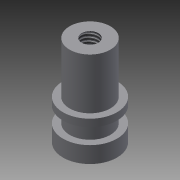
# Autodesk Inventor part: peek-insulator
Saved by Autodesk Inventor 2014 (Build 180170000, 170)
## iProperties
Created: 2013-12-31
Part Number: peek-insulator
Material: Generic
Document SubType Name: Modeling
Designer: caleb
Density: 1 g/cm^3
Appearance: Default
Author: caleb
Autodesk Inventor part; units mm, degrees
ref_plane "YZ Plane" through (0, 0, 0) normal (1, 0, 0) x (0, 1, 0)
ref_plane "XZ Plane" through (0, 0, 0) normal (0, 1, 0) x (-1, 0, 0)
ref_plane "XY Plane" through (0, 0, 0) normal (0, 0, 1) x (1, 0, 0)
sketch "Sketch1" plane through (0, 0, 0) normal (0, 0, 1) x (1, 0, 0)
  circle A0 centre (0, 0) radius 7.95
  dimension "d0" = 15.9
  constraints: 1 centre point, 1 coincident
  measures "d0" diameter of A0
extrude "Extrusion1" add sketch "Sketch1" along normal blind 4.82
sketch "Sketch2" plane through (0, 0, 4.82) normal (0, 0, 1) x (1, 0, 0)
  circle A0 centre (0, 0) radius 7.95 projected
  circle A1 centre (0, 0) radius 6
  dimension "d3" = 12
  constraints: 1 centre point, 1 coincident
  measures "d3" diameter of A1
extrude "Extrusion2" add sketch "Sketch2" along normal blind 4.6 contours A1
sketch "Sketch3" plane through (0, 0, 9.42) normal (0, 0, 1) x (1, 0, 0)
  circle A0 centre (0, 0) radius 6 projected
  circle A1 centre (0, 0) radius 7.95
  circle A2 centre (0, 0) radius 7.95 projected
  constraints: 1 centre point, 1 coincident, 1 concentric
extrude "Extrusion3" add sketch "Sketch3" along normal blind 2.15 contours A0 | A1
sketch "Sketch4" plane through (0, 0, 11.57) normal (0, 0, 1) x (1, 0, 0)
  circle A0 centre (0, 0) radius 7.95 projected
  circle A1 centre (0, 0) radius 6
  dimension "d8" = 12
  constraints: 1 centre point, 1 coincident
  measures "d8" diameter of A1
extrude "Extrusion4" add sketch "Sketch4" along normal blind 15 contours A1
sketch "Sketch5" plane through (0, 0, 0) normal (0, 0, -1) x (-1, 0, 0)
  circle A0 centre (0, 0) radius 7.95 projected
  constraints: 1 coincident
hole "Hole1" at (0, 0, 0) direction (0, 0, 1) diameter 4.917 end through all thread size "M6x1" class "6H" standard "ANSI Metric M Profile"
body "Solid1"
